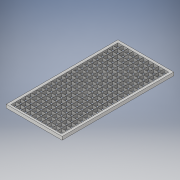
# Autodesk Inventor part: Lathhouse wall
Saved by Autodesk Inventor 2018 (Build 220112000, 112)
## iProperties
Created: 2019-05-08
Part Number: Lathhouse wall
Material: Generic
Document SubType Name: Modeling
Designer: 10043883
Density: 1 g/cm^3
Appearance: Default
Author: 10043883
Autodesk Inventor part; units mm, degrees
(part 1 of 2)
ref_plane "YZ Plane" through (0, 0, 0) normal (1, 0, 0) x (0, 1, 0)
ref_plane "XZ Plane" through (0, 0, 0) normal (0, 1, 0) x (-1, 0, 0)
ref_plane "XY Plane" through (0, 0, 0) normal (0, 0, 1) x (1, 0, 0)
sketch "Sketch1" plane through (0, 0, 0) normal (0, 1, 0) x (-1, 0, 0)
  line L0 (0, 0) -> (-3048, 0)
  line L1 (-3048, 0) -> (-3048, -6096)
  line L2 (-3048, -6096) -> (0, -6096)
  line L3 (0, -6096) -> (0, 0)
  dimension "d0" = 3048
  dimension "d1" = 6096
  constraints: 8 end point, 2 parallel, 1 horizontal, 1 perpendicular
  measures "d0" distance of L2.end L1.end
  measures "d1" distance of L1.end L0.end
extrude "Extrusion1" add sketch "Sketch1" along normal blind 177.8
sketch "Sketch2" plane through (0, 177.8, 0) normal (0, 1, 0) x (1, 0, 0)
  line L0 (146.7236, 110.4132) -> (400.7236, 110.4132)
  line L1 (400.7236, 110.4132) -> (400.7236, 364.4132)
  line L2 (400.7236, 364.4132) -> (146.7236, 364.4132)
  line L3 (146.7236, 364.4132) -> (146.7236, 110.4132)
  line L4 (146.7236, 110.4132) -> (400.7236, 364.4132) construction
  line L5 (400.7236, 110.4132) -> (146.7236, 364.4132) construction
  line L6 (400.7236, 110.4132) -> (3048, 110.4132) construction
  line L7 (3048, 0) -> (3048, 6096) construction
  line L8 (146.7236, 110.4132) -> (146.7236, 5658.2248) construction
  line L9 (146.7236, 389.8132) -> (400.7236, 389.8132)
  line L10 (400.7236, 389.8132) -> (400.7236, 643.8132)
  line L11 (400.7236, 643.8132) -> (146.7236, 643.8132)
  line L12 (146.7236, 643.8132) -> (146.7236, 389.8132)
  line L13 (146.7236, 669.2132) -> (400.7236, 669.2132)
  line L14 (400.7236, 669.2132) -> (400.7236, 923.2132)
  line L15 (400.7236, 923.2132) -> (146.7236, 923.2132)
  line L16 (146.7236, 923.2132) -> (146.7236, 669.2132)
  line L17 (146.7236, 948.6132) -> (400.7236, 948.6132)
  line L18 (400.7236, 948.6132) -> (400.7236, 1202.6132)
  line L19 (400.7236, 1202.6132) -> (146.7236, 1202.6132)
  line L20 (146.7236, 1202.6132) -> (146.7236, 948.6132)
  line L21 (146.7236, 1228.0132) -> (400.7236, 1228.0132)
  line L22 (400.7236, 1228.0132) -> (400.7236, 1482.0132)
  line L23 (400.7236, 1482.0132) -> (146.7236, 1482.0132)
  line L24 (146.7236, 1482.0132) -> (146.7236, 1228.0132)
  line L25 (146.7236, 1507.4132) -> (400.7236, 1507.4132)
  line L26 (400.7236, 1507.4132) -> (400.7236, 1761.4132)
  line L27 (400.7236, 1761.4132) -> (146.7236, 1761.4132)
  line L28 (146.7236, 1761.4132) -> (146.7236, 1507.4132)
  line L29 (146.7236, 1786.8132) -> (400.7236, 1786.8132)
  line L30 (400.7236, 1786.8132) -> (400.7236, 2040.8132)
  line L31 (400.7236, 2040.8132) -> (146.7236, 2040.8132)
  line L32 (146.7236, 2040.8132) -> (146.7236, 1786.8132)
  line L33 (146.7236, 2066.2132) -> (400.7236, 2066.2132)
  line L34 (400.7236, 2066.2132) -> (400.7236, 2320.2132)
  line L35 (400.7236, 2320.2132) -> (146.7236, 2320.2132)
  line L36 (146.7236, 2320.2132) -> (146.7236, 2066.2132)
  line L37 (146.7236, 2345.6132) -> (400.7236, 2345.6132)
  line L38 (400.7236, 2345.6132) -> (400.7236, 2599.6132)
  line L39 (400.7236, 2599.6132) -> (146.7236, 2599.6132)
  line L40 (146.7236, 2599.6132) -> (146.7236, 2345.6132)
  line L41 (146.7236, 2625.0132) -> (400.7236, 2625.0132)
  line L42 (400.7236, 2625.0132) -> (400.7236, 2879.0132)
  line L43 (400.7236, 2879.0132) -> (146.7236, 2879.0132)
  line L44 (146.7236, 2879.0132) -> (146.7236, 2625.0132)
  line L45 (146.7236, 2904.4132) -> (400.7236, 2904.4132)
  line L46 (400.7236, 2904.4132) -> (400.7236, 3158.4132)
  line L47 (400.7236, 3158.4132) -> (146.7236, 3158.4132)
  line L48 (146.7236, 3158.4132) -> (146.7236, 2904.4132)
  line L49 (146.7236, 3183.8132) -> (400.7236, 3183.8132)
  line L50 (400.7236, 3183.8132) -> (400.7236, 3437.8132)
  line L51 (400.7236, 3437.8132) -> (146.7236, 3437.8132)
  line L52 (146.7236, 3437.8132) -> (146.7236, 3183.8132)
  line L53 (146.7236, 3463.2132) -> (400.7236, 3463.2132)
  line L54 (400.7236, 3463.2132) -> (400.7236, 3717.2132)
  line L55 (400.7236, 3717.2132) -> (146.7236, 3717.2132)
  line L56 (146.7236, 3717.2132) -> (146.7236, 3463.2132)
  line L57 (146.7236, 3742.6132) -> (400.7236, 3742.6132)
  line L58 (400.7236, 3742.6132) -> (400.7236, 3996.6132)
  line L59 (400.7236, 3996.6132) -> (146.7236, 3996.6132)
  line L60 (146.7236, 3996.6132) -> (146.7236, 3742.6132)
  line L61 (146.7236, 4022.0132) -> (400.7236, 4022.0132)
  line L62 (400.7236, 4022.0132) -> (400.7236, 4276.0132)
  line L63 (400.7236, 4276.0132) -> (146.7236, 4276.0132)
  line L64 (146.7236, 4276.0132) -> (146.7236, 4022.0132)
  line L65 (146.7236, 4301.4132) -> (400.7236, 4301.4132)
  line L66 (400.7236, 4301.4132) -> (400.7236, 4555.4132)
  line L67 (400.7236, 4555.4132) -> (146.7236, 4555.4132)
  line L68 (146.7236, 4555.4132) -> (146.7236, 4301.4132)
  line L69 (146.7236, 4580.8132) -> (400.7236, 4580.8132)
  line L70 (400.7236, 4580.8132) -> (400.7236, 4834.8132)
  line L71 (400.7236, 4834.8132) -> (146.7236, 4834.8132)
  line L72 (146.7236, 4834.8132) -> (146.7236, 4580.8132)
  line L73 (146.7236, 4860.2132) -> (400.7236, 4860.2132)
  line L74 (400.7236, 4860.2132) -> (400.7236, 5114.2132)
  line L75 (400.7236, 5114.2132) -> (146.7236, 5114.2132)
  line L76 (146.7236, 5114.2132) -> (146.7236, 4860.2132)
  line L77 (146.7236, 5139.6132) -> (400.7236, 5139.6132)
  line L78 (400.7236, 5139.6132) -> (400.7236, 5393.6132)
  line L79 (400.7236, 5393.6132) -> (146.7236, 5393.6132)
  line L80 (146.7236, 5393.6132) -> (146.7236, 5139.6132)
  line L81 (146.7236, 5419.0132) -> (400.7236, 5419.0132)
  line L82 (400.7236, 5419.0132) -> (400.7236, 5673.0132)
  line L83 (400.7236, 5673.0132) -> (146.7236, 5673.0132)
  line L84 (146.7236, 5673.0132) -> (146.7236, 5419.0132)
  line L85 (146.7236, 5698.4132) -> (400.7236, 5698.4132)
  line L86 (400.7236, 5698.4132) -> (400.7236, 5952.4132)
  line L87 (400.7236, 5952.4132) -> (146.7236, 5952.4132)
  line L88 (146.7236, 5952.4132) -> (146.7236, 5698.4132)
  line L89 (426.1236, 110.4132) -> (680.1236, 110.4132)
  line L90 (680.1236, 110.4132) -> (680.1236, 364.4132)
  line L91 (680.1236, 364.4132) -> (426.1236, 364.4132)
  line L92 (426.1236, 364.4132) -> (426.1236, 110.4132)
  line L93 (426.1236, 389.8132) -> (680.1236, 389.8132)
  line L94 (680.1236, 389.8132) -> (680.1236, 643.8132)
  line L95 (680.1236, 643.8132) -> (426.1236, 643.8132)
  line L96 (426.1236, 643.8132) -> (426.1236, 389.8132)
  line L97 (426.1236, 669.2132) -> (680.1236, 669.2132)
  line L98 (680.1236, 669.2132) -> (680.1236, 923.2132)
  line L99 (680.1236, 923.2132) -> (426.1236, 923.2132)
  line L100 (426.1236, 923.2132) -> (426.1236, 669.2132)
  line L101 (426.1236, 948.6132) -> (680.1236, 948.6132)
  line L102 (680.1236, 948.6132) -> (680.1236, 1202.6132)
  line L103 (680.1236, 1202.6132) -> (426.1236, 1202.6132)
  line L104 (426.1236, 1202.6132) -> (426.1236, 948.6132)
  line L105 (426.1236, 1228.0132) -> (680.1236, 1228.0132)
  line L106 (680.1236, 1228.0132) -> (680.1236, 1482.0132)
  line L107 (680.1236, 1482.0132) -> (426.1236, 1482.0132)
  line L108 (426.1236, 1482.0132) -> (426.1236, 1228.0132)
  line L109 (426.1236, 1507.4132) -> (680.1236, 1507.4132)
  line L110 (680.1236, 1507.4132) -> (680.1236, 1761.4132)
  line L111 (680.1236, 1761.4132) -> (426.1236, 1761.4132)
  line L112 (426.1236, 1761.4132) -> (426.1236, 1507.4132)
  line L113 (426.1236, 1786.8132) -> (680.1236, 1786.8132)
  line L114 (680.1236, 1786.8132) -> (680.1236, 2040.8132)
  line L115 (680.1236, 2040.8132) -> (426.1236, 2040.8132)
  line L116 (426.1236, 2040.8132) -> (426.1236, 1786.8132)
  line L117 (426.1236, 2066.2132) -> (680.1236, 2066.2132)
  line L118 (680.1236, 2066.2132) -> (680.1236, 2320.2132)
  line L119 (680.1236, 2320.2132) -> (426.1236, 2320.2132)
  line L120 (426.1236, 2320.2132) -> (426.1236, 2066.2132)
  line L121 (426.1236, 2345.6132) -> (680.1236, 2345.6132)
  line L122 (680.1236, 2345.6132) -> (680.1236, 2599.6132)
  line L123 (680.1236, 2599.6132) -> (426.1236, 2599.6132)
  line L124 (426.1236, 2599.6132) -> (426.1236, 2345.6132)
  line L125 (426.1236, 2625.0132) -> (680.1236, 2625.0132)
  line L126 (680.1236, 2625.0132) -> (680.1236, 2879.0132)
  line L127 (680.1236, 2879.0132) -> (426.1236, 2879.0132)
  line L128 (426.1236, 2879.0132) -> (426.1236, 2625.0132)
  line L129 (426.1236, 2904.4132) -> (680.1236, 2904.4132)
  line L130 (680.1236, 2904.4132) -> (680.1236, 3158.4132)
  line L131 (680.1236, 3158.4132) -> (426.1236, 3158.4132)
  line L132 (426.1236, 3158.4132) -> (426.1236, 2904.4132)
  line L133 (426.1236, 3183.8132) -> (680.1236, 3183.8132)
  line L134 (680.1236, 3183.8132) -> (680.1236, 3437.8132)
  line L135 (680.1236, 3437.8132) -> (426.1236, 3437.8132)
  line L136 (426.1236, 3437.8132) -> (426.1236, 3183.8132)
  line L137 (426.1236, 3463.2132) -> (680.1236, 3463.2132)
  line L138 (680.1236, 3463.2132) -> (680.1236, 3717.2132)
  line L139 (680.1236, 3717.2132) -> (426.1236, 3717.2132)
  line L140 (426.1236, 3717.2132) -> (426.1236, 3463.2132)
  line L141 (426.1236, 3742.6132) -> (680.1236, 3742.6132)
  line L142 (680.1236, 3742.6132) -> (680.1236, 3996.6132)
  line L143 (680.1236, 3996.6132) -> (426.1236, 3996.6132)
  line L144 (426.1236, 3996.6132) -> (426.1236, 3742.6132)
  line L145 (426.1236, 4022.0132) -> (680.1236, 4022.0132)
  line L146 (680.1236, 4022.0132) -> (680.1236, 4276.0132)
  line L147 (680.1236, 4276.0132) -> (426.1236, 4276.0132)
  line L148 (426.1236, 4276.0132) -> (426.1236, 4022.0132)
  line L149 (426.1236, 4301.4132) -> (680.1236, 4301.4132)
  line L150 (680.1236, 4301.4132) -> (680.1236, 4555.4132)
  line L151 (680.1236, 4555.4132) -> (426.1236, 4555.4132)
  line L152 (426.1236, 4555.4132) -> (426.1236, 4301.4132)
  line L153 (426.1236, 4580.8132) -> (680.1236, 4580.8132)
  line L154 (680.1236, 4580.8132) -> (680.1236, 4834.8132)
  line L155 (680.1236, 4834.8132) -> (426.1236, 4834.8132)
  line L156 (426.1236, 4834.8132) -> (426.1236, 4580.8132)
  line L157 (426.1236, 4860.2132) -> (680.1236, 4860.2132)
  line L158 (680.1236, 4860.2132) -> (680.1236, 5114.2132)
  line L159 (680.1236, 5114.2132) -> (426.1236, 5114.2132)
  line L160 (426.1236, 5114.2132) -> (426.1236, 4860.2132)
  line L161 (426.1236, 5139.6132) -> (680.1236, 5139.6132)
  line L162 (680.1236, 5139.6132) -> (680.1236, 5393.6132)
  line L163 (680.1236, 5393.6132) -> (426.1236, 5393.6132)
  line L164 (426.1236, 5393.6132) -> (426.1236, 5139.6132)
  line L165 (426.1236, 5419.0132) -> (680.1236, 5419.0132)
  line L166 (680.1236, 5419.0132) -> (680.1236, 5673.0132)
  line L167 (680.1236, 5673.0132) -> (426.1236, 5673.0132)
  line L168 (426.1236, 5673.0132) -> (426.1236, 5419.0132)
  line L169 (426.1236, 5698.4132) -> (680.1236, 5698.4132)
  line L170 (680.1236, 5698.4132) -> (680.1236, 5952.4132)
  line L171 (680.1236, 5952.4132) -> (426.1236, 5952.4132)
  line L172 (426.1236, 5952.4132) -> (426.1236, 5698.4132)
  line L173 (705.5236, 110.4132) -> (959.5236, 110.4132)
  line L174 (959.5236, 110.4132) -> (959.5236, 364.4132)
  line L175 (959.5236, 364.4132) -> (705.5236, 364.4132)
  line L176 (705.5236, 364.4132) -> (705.5236, 110.4132)
  line L177 (705.5236, 389.8132) -> (959.5236, 389.8132)
  line L178 (959.5236, 389.8132) -> (959.5236, 643.8132)
  line L179 (959.5236, 643.8132) -> (705.5236, 643.8132)
  line L180 (705.5236, 643.8132) -> (705.5236, 389.8132)
  line L181 (705.5236, 669.2132) -> (959.5236, 669.2132)
  line L182 (959.5236, 669.2132) -> (959.5236, 923.2132)
  line L183 (959.5236, 923.2132) -> (705.5236, 923.2132)
  line L184 (705.5236, 923.2132) -> (705.5236, 669.2132)
  line L185 (705.5236, 948.6132) -> (959.5236, 948.6132)
  line L186 (959.5236, 948.6132) -> (959.5236, 1202.6132)
  line L187 (959.5236, 1202.6132) -> (705.5236, 1202.6132)
  line L188 (705.5236, 1202.6132) -> (705.5236, 948.6132)
  line L189 (705.5236, 1228.0132) -> (959.5236, 1228.0132)
  line L190 (959.5236, 1228.0132) -> (959.5236, 1482.0132)
  line L191 (959.5236, 1482.0132) -> (705.5236, 1482.0132)
  line L192 (705.5236, 1482.0132) -> (705.5236, 1228.0132)
  line L193 (705.5236, 1507.4132) -> (959.5236, 1507.4132)
  line L194 (959.5236, 1507.4132) -> (959.5236, 1761.4132)
  line L195 (959.5236, 1761.4132) -> (705.5236, 1761.4132)
  line L196 (705.5236, 1761.4132) -> (705.5236, 1507.4132)
  line L197 (705.5236, 1786.8132) -> (959.5236, 1786.8132)
  line L198 (959.5236, 1786.8132) -> (959.5236, 2040.8132)
  line L199 (959.5236, 2040.8132) -> (705.5236, 2040.8132)
  line L200 (705.5236, 2040.8132) -> (705.5236, 1786.8132)
  line L201 (705.5236, 2066.2132) -> (959.5236, 2066.2132)
  line L202 (959.5236, 2066.2132) -> (959.5236, 2320.2132)
  line L203 (959.5236, 2320.2132) -> (705.5236, 2320.2132)
  line L204 (705.5236, 2320.2132) -> (705.5236, 2066.2132)
  line L205 (705.5236, 2345.6132) -> (959.5236, 2345.6132)
  line L206 (959.5236, 2345.6132) -> (959.5236, 2599.6132)
  line L207 (959.5236, 2599.6132) -> (705.5236, 2599.6132)
  line L208 (705.5236, 2599.6132) -> (705.5236, 2345.6132)
  line L209 (705.5236, 2625.0132) -> (959.5236, 2625.0132)
  line L210 (959.5236, 2625.0132) -> (959.5236, 2879.0132)
  line L211 (959.5236, 2879.0132) -> (705.5236, 2879.0132)
  line L212 (705.5236, 2879.0132) -> (705.5236, 2625.0132)
  line L213 (705.5236, 2904.4132) -> (959.5236, 2904.4132)
  line L214 (959.5236, 2904.4132) -> (959.5236, 3158.4132)
  line L215 (959.5236, 3158.4132) -> (705.5236, 3158.4132)
  line L216 (705.5236, 3158.4132) -> (705.5236, 2904.4132)
  line L217 (705.5236, 3183.8132) -> (959.5236, 3183.8132)
  line L218 (959.5236, 3183.8132) -> (959.5236, 3437.8132)
  line L219 (959.5236, 3437.8132) -> (705.5236, 3437.8132)
  line L220 (705.5236, 3437.8132) -> (705.5236, 3183.8132)
  line L221 (705.5236, 3463.2132) -> (959.5236, 3463.2132)
  line L222 (959.5236, 3463.2132) -> (959.5236, 3717.2132)
  line L223 (959.5236, 3717.2132) -> (705.5236, 3717.2132)
  line L224 (705.5236, 3717.2132) -> (705.5236, 3463.2132)
  line L225 (705.5236, 3742.6132) -> (959.5236, 3742.6132)
  line L226 (959.5236, 3742.6132) -> (959.5236, 3996.6132)
  line L227 (959.5236, 3996.6132) -> (705.5236, 3996.6132)
  line L228 (705.5236, 3996.6132) -> (705.5236, 3742.6132)
  line L229 (705.5236, 4022.0132) -> (959.5236, 4022.0132)
  line L230 (959.5236, 4022.0132) -> (959.5236, 4276.0132)
  line L231 (959.5236, 4276.0132) -> (705.5236, 4276.0132)
  line L232 (705.5236, 4276.0132) -> (705.5236, 4022.0132)
  line L233 (705.5236, 4301.4132) -> (959.5236, 4301.4132)
  line L234 (959.5236, 4301.4132) -> (959.5236, 4555.4132)
  line L235 (959.5236, 4555.4132) -> (705.5236, 4555.4132)
  line L236 (705.5236, 4555.4132) -> (705.5236, 4301.4132)
  line L237 (705.5236, 4580.8132) -> (959.5236, 4580.8132)
  line L238 (959.5236, 4580.8132) -> (959.5236, 4834.8132)
  line L239 (959.5236, 4834.8132) -> (705.5236, 4834.8132)
  line L240 (705.5236, 4834.8132) -> (705.5236, 4580.8132)
  line L241 (705.5236, 4860.2132) -> (959.5236, 4860.2132)
  line L242 (959.5236, 4860.2132) -> (959.5236, 5114.2132)
  line L243 (959.5236, 5114.2132) -> (705.5236, 5114.2132)
  line L244 (705.5236, 5114.2132) -> (705.5236, 4860.2132)
  line L245 (705.5236, 5139.6132) -> (959.5236, 5139.6132)
  line L246 (959.5236, 5139.6132) -> (959.5236, 5393.6132)
  line L247 (959.5236, 5393.6132) -> (705.5236, 5393.6132)
  line L248 (705.5236, 5393.6132) -> (705.5236, 5139.6132)
  line L249 (705.5236, 5419.0132) -> (959.5236, 5419.0132)
  line L250 (959.5236, 5419.0132) -> (959.5236, 5673.0132)
  line L251 (959.5236, 5673.0132) -> (705.5236, 5673.0132)
  line L252 (705.5236, 5673.0132) -> (705.5236, 5419.0132)
  line L253 (705.5236, 5698.4132) -> (959.5236, 5698.4132)
  line L254 (959.5236, 5698.4132) -> (959.5236, 5952.4132)
  line L255 (959.5236, 5952.4132) -> (705.5236, 5952.4132)
  line L256 (705.5236, 5952.4132) -> (705.5236, 5698.4132)
  line L257 (984.9236, 110.4132) -> (1238.9236, 110.4132)
  line L258 (1238.9236, 110.4132) -> (1238.9236, 364.4132)
  line L259 (1238.9236, 364.4132) -> (984.9236, 364.4132)
  line L260 (984.9236, 364.4132) -> (984.9236, 110.4132)
  line L261 (984.9236, 389.8132) -> (1238.9236, 389.8132)
  line L262 (1238.9236, 389.8132) -> (1238.9236, 643.8132)
  line L263 (1238.9236, 643.8132) -> (984.9236, 643.8132)
  line L264 (984.9236, 643.8132) -> (984.9236, 389.8132)
  line L265 (984.9236, 669.2132) -> (1238.9236, 669.2132)
  line L266 (1238.9236, 669.2132) -> (1238.9236, 923.2132)
  line L267 (1238.9236, 923.2132) -> (984.9236, 923.2132)
  line L268 (984.9236, 923.2132) -> (984.9236, 669.2132)
  line L269 (984.9236, 948.6132) -> (1238.9236, 948.6132)
  line L270 (1238.9236, 948.6132) -> (1238.9236, 1202.6132)
  line L271 (1238.9236, 1202.6132) -> (984.9236, 1202.6132)
  line L272 (984.9236, 1202.6132) -> (984.9236, 948.6132)
  line L273 (984.9236, 1228.0132) -> (1238.9236, 1228.0132)
  line L274 (1238.9236, 1228.0132) -> (1238.9236, 1482.0132)
  line L275 (1238.9236, 1482.0132) -> (984.9236, 1482.0132)
  line L276 (984.9236, 1482.0132) -> (984.9236, 1228.0132)
  line L277 (984.9236, 1507.4132) -> (1238.9236, 1507.4132)
  line L278 (1238.9236, 1507.4132) -> (1238.9236, 1761.4132)
  line L279 (1238.9236, 1761.4132) -> (984.9236, 1761.4132)
  line L280 (984.9236, 1761.4132) -> (984.9236, 1507.4132)
  line L281 (984.9236, 1786.8132) -> (1238.9236, 1786.8132)
  line L282 (1238.9236, 1786.8132) -> (1238.9236, 2040.8132)
  line L283 (1238.9236, 2040.8132) -> (984.9236, 2040.8132)
  line L284 (984.9236, 2040.8132) -> (984.9236, 1786.8132)
  line L285 (984.9236, 2066.2132) -> (1238.9236, 2066.2132)
  line L286 (1238.9236, 2066.2132) -> (1238.9236, 2320.2132)
  line L287 (1238.9236, 2320.2132) -> (984.9236, 2320.2132)
  line L288 (984.9236, 2320.2132) -> (984.9236, 2066.2132)
  line L289 (984.9236, 2345.6132) -> (1238.9236, 2345.6132)
  line L290 (1238.9236, 2345.6132) -> (1238.9236, 2599.6132)
  line L291 (1238.9236, 2599.6132) -> (984.9236, 2599.6132)
  line L292 (984.9236, 2599.6132) -> (984.9236, 2345.6132)
  line L293 (984.9236, 2625.0132) -> (1238.9236, 2625.0132)
  line L294 (1238.9236, 2625.0132) -> (1238.9236, 2879.0132)
  line L295 (1238.9236, 2879.0132) -> (984.9236, 2879.0132)
  line L296 (984.9236, 2879.0132) -> (984.9236, 2625.0132)
  line L297 (984.9236, 2904.4132) -> (1238.9236, 2904.4132)
  line L298 (1238.9236, 2904.4132) -> (1238.9236, 3158.4132)
  line L299 (1238.9236, 3158.4132) -> (984.9236, 3158.4132)
  line L300 (984.9236, 3158.4132) -> (984.9236, 2904.4132)
  line L301 (984.9236, 3183.8132) -> (1238.9236, 3183.8132)
  line L302 (1238.9236, 3183.8132) -> (1238.9236, 3437.8132)
  line L303 (1238.9236, 3437.8132) -> (984.9236, 3437.8132)
  line L304 (984.9236, 3437.8132) -> (984.9236, 3183.8132)
  line L305 (984.9236, 3463.2132) -> (1238.9236, 3463.2132)
  line L306 (1238.9236, 3463.2132) -> (1238.9236, 3717.2132)
  line L307 (1238.9236, 3717.2132) -> (984.9236, 3717.2132)
  line L308 (984.9236, 3717.2132) -> (984.9236, 3463.2132)
  line L309 (984.9236, 3742.6132) -> (1238.9236, 3742.6132)
  line L310 (1238.9236, 3742.6132) -> (1238.9236, 3996.6132)
  line L311 (1238.9236, 3996.6132) -> (984.9236, 3996.6132)
  line L312 (984.9236, 3996.6132) -> (984.9236, 3742.6132)
  line L313 (984.9236, 4022.0132) -> (1238.9236, 4022.0132)
  line L314 (1238.9236, 4022.0132) -> (1238.9236, 4276.0132)
  line L315 (1238.9236, 4276.0132) -> (984.9236, 4276.0132)
  line L316 (984.9236, 4276.0132) -> (984.9236, 4022.0132)
  line L317 (984.9236, 4301.4132) -> (1238.9236, 4301.4132)
  line L318 (1238.9236, 4301.4132) -> (1238.9236, 4555.4132)
  line L319 (1238.9236, 4555.4132) -> (984.9236, 4555.4132)
  line L320 (984.9236, 4555.4132) -> (984.9236, 4301.4132)
  line L321 (984.9236, 4580.8132) -> (1238.9236, 4580.8132)
  line L322 (1238.9236, 4580.8132) -> (1238.9236, 4834.8132)
  line L323 (1238.9236, 4834.8132) -> (984.9236, 4834.8132)
  line L324 (984.9236, 4834.8132) -> (984.9236, 4580.8132)
  line L325 (984.9236, 4860.2132) -> (1238.9236, 4860.2132)
  line L326 (1238.9236, 4860.2132) -> (1238.9236, 5114.2132)
  line L327 (1238.9236, 5114.2132) -> (984.9236, 5114.2132)
  line L328 (984.9236, 5114.2132) -> (984.9236, 4860.2132)
  line L329 (984.9236, 5139.6132) -> (1238.9236, 5139.6132)
  line L330 (1238.9236, 5139.6132) -> (1238.9236, 5393.6132)
  line L331 (1238.9236, 5393.6132) -> (984.9236, 5393.6132)
  line L332 (984.9236, 5393.6132) -> (984.9236, 5139.6132)
  line L333 (984.9236, 5419.0132) -> (1238.9236, 5419.0132)
  line L334 (1238.9236, 5419.0132) -> (1238.9236, 5673.0132)
  line L335 (1238.9236, 5673.0132) -> (984.9236, 5673.0132)
  line L336 (984.9236, 5673.0132) -> (984.9236, 5419.0132)
  line L337 (984.9236, 5698.4132) -> (1238.9236, 5698.4132)
  line L338 (1238.9236, 5698.4132) -> (1238.9236, 5952.4132)
  line L339 (1238.9236, 5952.4132) -> (984.9236, 5952.4132)
  line L340 (984.9236, 5952.4132) -> (984.9236, 5698.4132)
  line L341 (1264.3236, 110.4132) -> (1518.3236, 110.4132)
  line L342 (1518.3236, 110.4132) -> (1518.3236, 364.4132)
  line L343 (1518.3236, 364.4132) -> (1264.3236, 364.4132)
  line L344 (1264.3236, 364.4132) -> (1264.3236, 110.4132)
  line L345 (1264.3236, 389.8132) -> (1518.3236, 389.8132)
  line L346 (1518.3236, 389.8132) -> (1518.3236, 643.8132)
  line L347 (1518.3236, 643.8132) -> (1264.3236, 643.8132)
  line L348 (1264.3236, 643.8132) -> (1264.3236, 389.8132)
  line L349 (1264.3236, 669.2132) -> (1518.3236, 669.2132)
  line L350 (1518.3236, 669.2132) -> (1518.3236, 923.2132)
  line L351 (1518.3236, 923.2132) -> (1264.3236, 923.2132)
  line L352 (1264.3236, 923.2132) -> (1264.3236, 669.2132)
  line L353 (1264.3236, 948.6132) -> (1518.3236, 948.6132)
  line L354 (1518.3236, 948.6132) -> (1518.3236, 1202.6132)
  line L355 (1518.3236, 1202.6132) -> (1264.3236, 1202.6132)
  line L356 (1264.3236, 1202.6132) -> (1264.3236, 948.6132)
  line L357 (1264.3236, 1228.0132) -> (1518.3236, 1228.0132)
  line L358 (1518.3236, 1228.0132) -> (1518.3236, 1482.0132)
  line L359 (1518.3236, 1482.0132) -> (1264.3236, 1482.0132)
  line L360 (1264.3236, 1482.0132) -> (1264.3236, 1228.0132)
  line L361 (1264.3236, 1507.4132) -> (1518.3236, 1507.4132)
  line L362 (1518.3236, 1507.4132) -> (1518.3236, 1761.4132)
  line L363 (1518.3236, 1761.4132) -> (1264.3236, 1761.4132)
  line L364 (1264.3236, 1761.4132) -> (1264.3236, 1507.4132)
  line L365 (1264.3236, 1786.8132) -> (1518.3236, 1786.8132)
  line L366 (1518.3236, 1786.8132) -> (1518.3236, 2040.8132)
  line L367 (1518.3236, 2040.8132) -> (1264.3236, 2040.8132)
  line L368 (1264.3236, 2040.8132) -> (1264.3236, 1786.8132)
  line L369 (1264.3236, 2066.2132) -> (1518.3236, 2066.2132)
  line L370 (1518.3236, 2066.2132) -> (1518.3236, 2320.2132)
  line L371 (1518.3236, 2320.2132) -> (1264.3236, 2320.2132)
  line L372 (1264.3236, 2320.2132) -> (1264.3236, 2066.2132)
  line L373 (1264.3236, 2345.6132) -> (1518.3236, 2345.6132)
  line L374 (1518.3236, 2345.6132) -> (1518.3236, 2599.6132)
  line L375 (1518.3236, 2599.6132) -> (1264.3236, 2599.6132)
  line L376 (1264.3236, 2599.6132) -> (1264.3236, 2345.6132)
  line L377 (1264.3236, 2625.0132) -> (1518.3236, 2625.0132)
  line L378 (1518.3236, 2625.0132) -> (1518.3236, 2879.0132)
  line L379 (1518.3236, 2879.0132) -> (1264.3236, 2879.0132)
  line L380 (1264.3236, 2879.0132) -> (1264.3236, 2625.0132)
  line L381 (1264.3236, 2904.4132) -> (1518.3236, 2904.4132)
  line L382 (1518.3236, 2904.4132) -> (1518.3236, 3158.4132)
  line L383 (1518.3236, 3158.4132) -> (1264.3236, 3158.4132)
  line L384 (1264.3236, 3158.4132) -> (1264.3236, 2904.4132)
  line L385 (1264.3236, 3183.8132) -> (1518.3236, 3183.8132)
  line L386 (1518.3236, 3183.8132) -> (1518.3236, 3437.8132)
  line L387 (1518.3236, 3437.8132) -> (1264.3236, 3437.8132)
  line L388 (1264.3236, 3437.8132) -> (1264.3236, 3183.8132)
  line L389 (1264.3236, 3463.2132) -> (1518.3236, 3463.2132)
  line L390 (1518.3236, 3463.2132) -> (1518.3236, 3717.2132)
  line L391 (1518.3236, 3717.2132) -> (1264.3236, 3717.2132)
  line L392 (1264.3236, 3717.2132) -> (1264.3236, 3463.2132)
  line L393 (1264.3236, 3742.6132) -> (1518.3236, 3742.6132)
  line L394 (1518.3236, 3742.6132) -> (1518.3236, 3996.6132)
  line L395 (1518.3236, 3996.6132) -> (1264.3236, 3996.6132)
  line L396 (1264.3236, 3996.6132) -> (1264.3236, 3742.6132)
  line L397 (1264.3236, 4022.0132) -> (1518.3236, 4022.0132)
  line L398 (1518.3236, 4022.0132) -> (1518.3236, 4276.0132)
  line L399 (1518.3236, 4276.0132) -> (1264.3236, 4276.0132)
  line L400 (1264.3236, 4276.0132) -> (1264.3236, 4022.0132)
  line L401 (1264.3236, 4301.4132) -> (1518.3236, 4301.4132)
  line L402 (1518.3236, 4301.4132) -> (1518.3236, 4555.4132)
  line L403 (1518.3236, 4555.4132) -> (1264.3236, 4555.4132)
  line L404 (1264.3236, 4555.4132) -> (1264.3236, 4301.4132)
  line L405 (1264.3236, 4580.8132) -> (1518.3236, 4580.8132)
  line L406 (1518.3236, 4580.8132) -> (1518.3236, 4834.8132)
  line L407 (1518.3236, 4834.8132) -> (1264.3236, 4834.8132)
  line L408 (1264.3236, 4834.8132) -> (1264.3236, 4580.8132)
  line L409 (1264.3236, 4860.2132) -> (1518.3236, 4860.2132)
  line L410 (1518.3236, 4860.2132) -> (1518.3236, 5114.2132)
  line L411 (1518.3236, 5114.2132) -> (1264.3236, 5114.2132)
  line L412 (1264.3236, 5114.2132) -> (1264.3236, 4860.2132)
  line L413 (1264.3236, 5139.6132) -> (1518.3236, 5139.6132)
  line L414 (1518.3236, 5139.6132) -> (1518.3236, 5393.6132)
  line L415 (1518.3236, 5393.6132) -> (1264.3236, 5393.6132)
  line L416 (1264.3236, 5393.6132) -> (1264.3236, 5139.6132)
  line L417 (1264.3236, 5419.0132) -> (1518.3236, 5419.0132)
  line L418 (1518.3236, 5419.0132) -> (1518.3236, 5673.0132)
  line L419 (1518.3236, 5673.0132) -> (1264.3236, 5673.0132)
  line L420 (1264.3236, 5673.0132) -> (1264.3236, 5419.0132)
  line L421 (1264.3236, 5698.4132) -> (1518.3236, 5698.4132)
  line L422 (1518.3236, 5698.4132) -> (1518.3236, 5952.4132)
  line L423 (1518.3236, 5952.4132) -> (1264.3236, 5952.4132)
  line L424 (1264.3236, 5952.4132) -> (1264.3236, 5698.4132)
  line L425 (1543.7236, 110.4132) -> (1797.7236, 110.4132)
  line L426 (1797.7236, 110.4132) -> (1797.7236, 364.4132)
  line L427 (1797.7236, 364.4132) -> (1543.7236, 364.4132)
  line L428 (1543.7236, 364.4132) -> (1543.7236, 110.4132)
  line L429 (1543.7236, 389.8132) -> (1797.7236, 389.8132)
  line L430 (1797.7236, 389.8132) -> (1797.7236, 643.8132)
  line L431 (1797.7236, 643.8132) -> (1543.7236, 643.8132)
  line L432 (1543.7236, 643.8132) -> (1543.7236, 389.8132)
  line L433 (1543.7236, 669.2132) -> (1797.7236, 669.2132)
  line L434 (1797.7236, 669.2132) -> (1797.7236, 923.2132)
  line L435 (1797.7236, 923.2132) -> (1543.7236, 923.2132)
  line L436 (1543.7236, 923.2132) -> (1543.7236, 669.2132)
  line L437 (1543.7236, 948.6132) -> (1797.7236, 948.6132)
  line L438 (1797.7236, 948.6132) -> (1797.7236, 1202.6132)
  line L439 (1797.7236, 1202.6132) -> (1543.7236, 1202.6132)
  line L440 (1543.7236, 1202.6132) -> (1543.7236, 948.6132)
  line L441 (1543.7236, 1228.0132) -> (1797.7236, 1228.0132)
  line L442 (1797.7236, 1228.0132) -> (1797.7236, 1482.0132)
  line L443 (1797.7236, 1482.0132) -> (1543.7236, 1482.0132)
  line L444 (1543.7236, 1482.0132) -> (1543.7236, 1228.0132)
  line L445 (1543.7236, 1507.4132) -> (1797.7236, 1507.4132)
  line L446 (1797.7236, 1507.4132) -> (1797.7236, 1761.4132)
  line L447 (1797.7236, 1761.4132) -> (1543.7236, 1761.4132)
  line L448 (1543.7236, 1761.4132) -> (1543.7236, 1507.4132)
  line L449 (1543.7236, 1786.8132) -> (1797.7236, 1786.8132)
  line L450 (1797.7236, 1786.8132) -> (1797.7236, 2040.8132)
  line L451 (1797.7236, 2040.8132) -> (1543.7236, 2040.8132)
  line L452 (1543.7236, 2040.8132) -> (1543.7236, 1786.8132)
  line L453 (1543.7236, 2066.2132) -> (1797.7236, 2066.2132)
  line L454 (1797.7236, 2066.2132) -> (1797.7236, 2320.2132)
  line L455 (1797.7236, 2320.2132) -> (1543.7236, 2320.2132)
  line L456 (1543.7236, 2320.2132) -> (1543.7236, 2066.2132)
  line L457 (1543.7236, 2345.6132) -> (1797.7236, 2345.6132)
  line L458 (1797.7236, 2345.6132) -> (1797.7236, 2599.6132)
  line L459 (1797.7236, 2599.6132) -> (1543.7236, 2599.6132)
  line L460 (1543.7236, 2599.6132) -> (1543.7236, 2345.6132)
  line L461 (1543.7236, 2625.0132) -> (1797.7236, 2625.0132)
  line L462 (1797.7236, 2625.0132) -> (1797.7236, 2879.0132)
  line L463 (1797.7236, 2879.0132) -> (1543.7236, 2879.0132)
  line L464 (1543.7236, 2879.0132) -> (1543.7236, 2625.0132)
  line L465 (1543.7236, 2904.4132) -> (1797.7236, 2904.4132)
  line L466 (1797.7236, 2904.4132) -> (1797.7236, 3158.4132)
  line L467 (1797.7236, 3158.4132) -> (1543.7236, 3158.4132)
  line L468 (1543.7236, 3158.4132) -> (1543.7236, 2904.4132)
  line L469 (1543.7236, 3183.8132) -> (1797.7236, 3183.8132)
  line L470 (1797.7236, 3183.8132) -> (1797.7236, 3437.8132)
  line L471 (1797.7236, 3437.8132) -> (1543.7236, 3437.8132)
  line L472 (1543.7236, 3437.8132) -> (1543.7236, 3183.8132)
  line L473 (1543.7236, 3463.2132) -> (1797.7236, 3463.2132)
  line L474 (1797.7236, 3463.2132) -> (1797.7236, 3717.2132)
  line L475 (1797.7236, 3717.2132) -> (1543.7236, 3717.2132)
  line L476 (1543.7236, 3717.2132) -> (1543.7236, 3463.2132)
  line L477 (1543.7236, 3742.6132) -> (1797.7236, 3742.6132)
  line L478 (1797.7236, 3742.6132) -> (1797.7236, 3996.6132)
  line L479 (1797.7236, 3996.6132) -> (1543.7236, 3996.6132)
  line L480 (1543.7236, 3996.6132) -> (1543.7236, 3742.6132)
  line L481 (1543.7236, 4022.0132) -> (1797.7236, 4022.0132)
  line L482 (1797.7236, 4022.0132) -> (1797.7236, 4276.0132)
  line L483 (1797.7236, 4276.0132) -> (1543.7236, 4276.0132)
  line L484 (1543.7236, 4276.0132) -> (1543.7236, 4022.0132)
  line L485 (1543.7236, 4301.4132) -> (1797.7236, 4301.4132)
  line L486 (1797.7236, 4301.4132) -> (1797.7236, 4555.4132)
  line L487 (1797.7236, 4555.4132) -> (1543.7236, 4555.4132)
  line L488 (1543.7236, 4555.4132) -> (1543.7236, 4301.4132)
  line L489 (1543.7236, 4580.8132) -> (1797.7236, 4580.8132)
  line L490 (1797.7236, 4580.8132) -> (1797.7236, 4834.8132)
  line L491 (1797.7236, 4834.8132) -> (1543.7236, 4834.8132)
  line L492 (1543.7236, 4834.8132) -> (1543.7236, 4580.8132)
  line L493 (1543.7236, 4860.2132) -> (1797.7236, 4860.2132)
  line L494 (1797.7236, 4860.2132) -> (1797.7236, 5114.2132)
  line L495 (1797.7236, 5114.2132) -> (1543.7236, 5114.2132)
  line L496 (1543.7236, 5114.2132) -> (1543.7236, 4860.2132)
  line L497 (1543.7236, 5139.6132) -> (1797.7236, 5139.6132)
  line L498 (1797.7236, 5139.6132) -> (1797.7236, 5393.6132)
  line L499 (1797.7236, 5393.6132) -> (1543.7236, 5393.6132)
  line L500 (1543.7236, 5393.6132) -> (1543.7236, 5139.6132)
  line L501 (1543.7236, 5419.0132) -> (1797.7236, 5419.0132)
  line L502 (1797.7236, 5419.0132) -> (1797.7236, 5673.0132)
  line L503 (1797.7236, 5673.0132) -> (1543.7236, 5673.0132)
  line L504 (1543.7236, 5673.0132) -> (1543.7236, 5419.0132)
  line L505 (1543.7236, 5698.4132) -> (1797.7236, 5698.4132)
  line L506 (1797.7236, 5698.4132) -> (1797.7236, 5952.4132)
  line L507 (1797.7236, 5952.4132) -> (1543.7236, 5952.4132)
  line L508 (1543.7236, 5952.4132) -> (1543.7236, 5698.4132)
  line L509 (1823.1236, 110.4132) -> (2077.1236, 110.4132)
  line L510 (2077.1236, 110.4132) -> (2077.1236, 364.4132)
  line L511 (2077.1236, 364.4132) -> (1823.1236, 364.4132)
  line L512 (1823.1236, 364.4132) -> (1823.1236, 110.4132)
  line L513 (1823.1236, 389.8132) -> (2077.1236, 389.8132)
  line L514 (2077.1236, 389.8132) -> (2077.1236, 643.8132)
  line L515 (2077.1236, 643.8132) -> (1823.1236, 643.8132)
  line L516 (1823.1236, 643.8132) -> (1823.1236, 389.8132)
  line L517 (1823.1236, 669.2132) -> (2077.1236, 669.2132)
  line L518 (2077.1236, 669.2132) -> (2077.1236, 923.2132)
  line L519 (2077.1236, 923.2132) -> (1823.1236, 923.2132)
  line L520 (1823.1236, 923.2132) -> (1823.1236, 669.2132)
  line L521 (1823.1236, 948.6132) -> (2077.1236, 948.6132)
  line L522 (2077.1236, 948.6132) -> (2077.1236, 1202.6132)
  line L523 (2077.1236, 1202.6132) -> (1823.1236, 1202.6132)
  line L524 (1823.1236, 1202.6132) -> (1823.1236, 948.6132)
  line L525 (1823.1236, 1228.0132) -> (2077.1236, 1228.0132)
  line L526 (2077.1236, 1228.0132) -> (2077.1236, 1482.0132)
  line L527 (2077.1236, 1482.0132) -> (1823.1236, 1482.0132)
  line L528 (1823.1236, 1482.0132) -> (1823.1236, 1228.0132)
  line L529 (1823.1236, 1507.4132) -> (2077.1236, 1507.4132)
  line L530 (2077.1236, 1507.4132) -> (2077.1236, 1761.4132)
  line L531 (2077.1236, 1761.4132) -> (1823.1236, 1761.4132)
  line L532 (1823.1236, 1761.4132) -> (1823.1236, 1507.4132)
  line L533 (1823.1236, 1786.8132) -> (2077.1236, 1786.8132)
  line L534 (2077.1236, 1786.8132) -> (2077.1236, 2040.8132)
  line L535 (2077.1236, 2040.8132) -> (1823.1236, 2040.8132)
  line L536 (1823.1236, 2040.8132) -> (1823.1236, 1786.8132)
  line L537 (1823.1236, 2066.2132) -> (2077.1236, 2066.2132)
  line L538 (2077.1236, 2066.2132) -> (2077.1236, 2320.2132)
  line L539 (2077.1236, 2320.2132) -> (1823.1236, 2320.2132)
  line L540 (1823.1236, 2320.2132) -> (1823.1236, 2066.2132)
  line L541 (1823.1236, 2345.6132) -> (2077.1236, 2345.6132)
  line L542 (2077.1236, 2345.6132) -> (2077.1236, 2599.6132)
  line L543 (2077.1236, 2599.6132) -> (1823.1236, 2599.6132)
  line L544 (1823.1236, 2599.6132) -> (1823.1236, 2345.6132)
  line L545 (1823.1236, 2625.0132) -> (2077.1236, 2625.0132)
  line L546 (2077.1236, 2625.0132) -> (2077.1236, 2879.0132)
  line L547 (2077.1236, 2879.0132) -> (1823.1236, 2879.0132)
  line L548 (1823.1236, 2879.0132) -> (1823.1236, 2625.0132)
  line L549 (1823.1236, 2904.4132) -> (2077.1236, 2904.4132)
  line L550 (2077.1236, 2904.4132) -> (2077.1236, 3158.4132)
  line L551 (2077.1236, 3158.4132) -> (1823.1236, 3158.4132)
  line L552 (1823.1236, 3158.4132) -> (1823.1236, 2904.4132)
  line L553 (1823.1236, 3183.8132) -> (2077.1236, 3183.8132)
  line L554 (2077.1236, 3183.8132) -> (2077.1236, 3437.8132)
  line L555 (2077.1236, 3437.8132) -> (1823.1236, 3437.8132)
  line L556 (1823.1236, 3437.8132) -> (1823.1236, 3183.8132)
  line L557 (1823.1236, 3463.2132) -> (2077.1236, 3463.2132)
  line L558 (2077.1236, 3463.2132) -> (2077.1236, 3717.2132)
  line L559 (2077.1236, 3717.2132) -> (1823.1236, 3717.2132)
  line L560 (1823.1236, 3717.2132) -> (1823.1236, 3463.2132)
  line L561 (1823.1236, 3742.6132) -> (2077.1236, 3742.6132)
  line L562 (2077.1236, 3742.6132) -> (2077.1236, 3996.6132)
  line L563 (2077.1236, 3996.6132) -> (1823.1236, 3996.6132)
  line L564 (1823.1236, 3996.6132) -> (1823.1236, 3742.6132)
  line L565 (1823.1236, 4022.0132) -> (2077.1236, 4022.0132)
  line L566 (2077.1236, 4022.0132) -> (2077.1236, 4276.0132)
  line L567 (2077.1236, 4276.0132) -> (1823.1236, 4276.0132)
  line L568 (1823.1236, 4276.0132) -> (1823.1236, 4022.0132)
  line L569 (1823.1236, 4301.4132) -> (2077.1236, 4301.4132)
  line L570 (2077.1236, 4301.4132) -> (2077.1236, 4555.4132)
  line L571 (2077.1236, 4555.4132) -> (1823.1236, 4555.4132)
  line L572 (1823.1236, 4555.4132) -> (1823.1236, 4301.4132)
  line L573 (1823.1236, 4580.8132) -> (2077.1236, 4580.8132)
  line L574 (2077.1236, 4580.8132) -> (2077.1236, 4834.8132)
  line L575 (2077.1236, 4834.8132) -> (1823.1236, 4834.8132)
  line L576 (1823.1236, 4834.8132) -> (1823.1236, 4580.8132)
  line L577 (1823.1236, 4860.2132) -> (2077.1236, 4860.2132)
  line L578 (2077.1236, 4860.2132) -> (2077.1236, 5114.2132)
  line L579 (2077.1236, 5114.2132) -> (1823.1236, 5114.2132)
  line L580 (1823.1236, 5114.2132) -> (1823.1236, 4860.2132)
  line L581 (1823.1236, 5139.6132) -> (2077.1236, 5139.6132)
  line L582 (2077.1236, 5139.6132) -> (2077.1236, 5393.6132)
  line L583 (2077.1236, 5393.6132) -> (1823.1236, 5393.6132)
  line L584 (1823.1236, 5393.6132) -> (1823.1236, 5139.6132)
  line L585 (1823.1236, 5419.0132) -> (2077.1236, 5419.0132)
  line L586 (2077.1236, 5419.0132) -> (2077.1236, 5673.0132)
  line L587 (2077.1236, 5673.0132) -> (1823.1236, 5673.0132)
  line L588 (1823.1236, 5673.0132) -> (1823.1236, 5419.0132)
  line L589 (1823.1236, 5698.4132) -> (2077.1236, 5698.4132)
  line L590 (2077.1236, 5698.4132) -> (2077.1236, 5952.4132)
  line L591 (2077.1236, 5952.4132) -> (1823.1236, 5952.4132)
  line L592 (1823.1236, 5952.4132) -> (1823.1236, 5698.4132)
  line L593 (2102.5236, 110.4132) -> (2356.5236, 110.4132)
  line L594 (2356.5236, 110.4132) -> (2356.5236, 364.4132)
  line L595 (2356.5236, 364.4132) -> (2102.5236, 364.4132)
  line L596 (2102.5236, 364.4132) -> (2102.5236, 110.4132)
  line L597 (2102.5236, 389.8132) -> (2356.5236, 389.8132)
  line L598 (2356.5236, 389.8132) -> (2356.5236, 643.8132)
  line L599 (2356.5236, 643.8132) -> (2102.5236, 643.8132)
  line L600 (2102.5236, 643.8132) -> (2102.5236, 389.8132)
  line L601 (2102.5236, 669.2132) -> (2356.5236, 669.2132)
  line L602 (2356.5236, 669.2132) -> (2356.5236, 923.2132)
  line L603 (2356.5236, 923.2132) -> (2102.5236, 923.2132)
  line L604 (2102.5236, 923.2132) -> (2102.5236, 669.2132)
  line L605 (2102.5236, 948.6132) -> (2356.5236, 948.6132)
  line L606 (2356.5236, 948.6132) -> (2356.5236, 1202.6132)
  line L607 (2356.5236, 1202.6132) -> (2102.5236, 1202.6132)
  line L608 (2102.5236, 1202.6132) -> (2102.5236, 948.6132)
  line L609 (2102.5236, 1228.0132) -> (2356.5236, 1228.0132)
  line L610 (2356.5236, 1228.0132) -> (2356.5236, 1482.0132)
  line L611 (2356.5236, 1482.0132) -> (2102.5236, 1482.0132)
  line L612 (2102.5236, 1482.0132) -> (2102.5236, 1228.0132)
  line L613 (2102.5236, 1507.4132) -> (2356.5236, 1507.4132)
  line L614 (2356.5236, 1507.4132) -> (2356.5236, 1761.4132)
  line L615 (2356.5236, 1761.4132) -> (2102.5236, 1761.4132)
  line L616 (2102.5236, 1761.4132) -> (2102.5236, 1507.4132)
  line L617 (2102.5236, 1786.8132) -> (2356.5236, 1786.8132)
  line L618 (2356.5236, 1786.8132) -> (2356.5236, 2040.8132)
  line L619 (2356.5236, 2040.8132) -> (2102.5236, 2040.8132)
  line L620 (2102.5236, 2040.8132) -> (2102.5236, 1786.8132)
  line L621 (2102.5236, 2066.2132) -> (2356.5236, 2066.2132)
  line L622 (2356.5236, 2066.2132) -> (2356.5236, 2320.2132)
  line L623 (2356.5236, 2320.2132) -> (2102.5236, 2320.2132)
  line L624 (2102.5236, 2320.2132) -> (2102.5236, 2066.2132)
  line L625 (2102.5236, 2345.6132) -> (2356.5236, 2345.6132)
  line L626 (2356.5236, 2345.6132) -> (2356.5236, 2599.6132)
  line L627 (2356.5236, 2599.6132) -> (2102.5236, 2599.6132)
  line L628 (2102.5236, 2599.6132) -> (2102.5236, 2345.6132)
  line L629 (2102.5236, 2625.0132) -> (2356.5236, 2625.0132)
  line L630 (2356.5236, 2625.0132) -> (2356.5236, 2879.0132)
  line L631 (2356.5236, 2879.0132) -> (2102.5236, 2879.0132)
  line L632 (2102.5236, 2879.0132) -> (2102.5236, 2625.0132)
  line L633 (2102.5236, 2904.4132) -> (2356.5236, 2904.4132)
  line L634 (2356.5236, 2904.4132) -> (2356.5236, 3158.4132)
  line L635 (2356.5236, 3158.4132) -> (2102.5236, 3158.4132)
  line L636 (2102.5236, 3158.4132) -> (2102.5236, 2904.4132)
  line L637 (2102.5236, 3183.8132) -> (2356.5236, 3183.8132)
  line L638 (2356.5236, 3183.8132) -> (2356.5236, 3437.8132)
  line L639 (2356.5236, 3437.8132) -> (2102.5236, 3437.8132)
  line L640 (2102.5236, 3437.8132) -> (2102.5236, 3183.8132)
  line L641 (2102.5236, 3463.2132) -> (2356.5236, 3463.2132)
  line L642 (2356.5236, 3463.2132) -> (2356.5236, 3717.2132)
  line L643 (2356.5236, 3717.2132) -> (2102.5236, 3717.2132)
  line L644 (2102.5236, 3717.2132) -> (2102.5236, 3463.2132)
  line L645 (2102.5236, 3742.6132) -> (2356.5236, 3742.6132)
  line L646 (2356.5236, 3742.6132) -> (2356.5236, 3996.6132)
  line L647 (2356.5236, 3996.6132) -> (2102.5236, 3996.6132)
  line L648 (2102.5236, 3996.6132) -> (2102.5236, 3742.6132)
  line L649 (2102.5236, 4022.0132) -> (2356.5236, 4022.0132)
  line L650 (2356.5236, 4022.0132) -> (2356.5236, 4276.0132)
  line L651 (2356.5236, 4276.0132) -> (2102.5236, 4276.0132)
  line L652 (2102.5236, 4276.0132) -> (2102.5236, 4022.0132)
  line L653 (2102.5236, 4301.4132) -> (2356.5236, 4301.4132)
  line L654 (2356.5236, 4301.4132) -> (2356.5236, 4555.4132)
  line L655 (2356.5236, 4555.4132) -> (2102.5236, 4555.4132)
  line L656 (2102.5236, 4555.4132) -> (2102.5236, 4301.4132)
  line L657 (2102.5236, 4580.8132) -> (2356.5236, 4580.8132)
  line L658 (2356.5236, 4580.8132) -> (2356.5236, 4834.8132)
  line L659 (2356.5236, 4834.8132) -> (2102.5236, 4834.8132)
  line L660 (2102.5236, 4834.8132) -> (2102.5236, 4580.8132)
  line L661 (2102.5236, 4860.2132) -> (2356.5236, 4860.2132)
  line L662 (2356.5236, 4860.2132) -> (2356.5236, 5114.2132)
  line L663 (2356.5236, 5114.2132) -> (2102.5236, 5114.2132)
  line L664 (2102.5236, 5114.2132) -> (2102.5236, 4860.2132)
  line L665 (2102.5236, 5139.6132) -> (2356.5236, 5139.6132)
  line L666 (2356.5236, 5139.6132) -> (2356.5236, 5393.6132)
  line L667 (2356.5236, 5393.6132) -> (2102.5236, 5393.6132)
  line L668 (2102.5236, 5393.6132) -> (2102.5236, 5139.6132)
  line L669 (2102.5236, 5419.0132) -> (2356.5236, 5419.0132)
  line L670 (2356.5236, 5419.0132) -> (2356.5236, 5673.0132)
  line L671 (2356.5236, 5673.0132) -> (2102.5236, 5673.0132)
  line L672 (2102.5236, 5673.0132) -> (2102.5236, 5419.0132)
  line L673 (2102.5236, 5698.4132) -> (2356.5236, 5698.4132)
  line L674 (2356.5236, 5698.4132) -> (2356.5236, 5952.4132)
  line L675 (2356.5236, 5952.4132) -> (2102.5236, 5952.4132)
  line L676 (2102.5236, 5952.4132) -> (2102.5236, 5698.4132)
  line L677 (2381.9236, 110.4132) -> (2635.9236, 110.4132)
  line L678 (2635.9236, 110.4132) -> (2635.9236, 364.4132)
  line L679 (2635.9236, 364.4132) -> (2381.9236, 364.4132)
  line L680 (2381.9236, 364.4132) -> (2381.9236, 110.4132)
  line L681 (2381.9236, 389.8132) -> (2635.9236, 389.8132)
  line L682 (2635.9236, 389.8132) -> (2635.9236, 643.8132)
  line L683 (2635.9236, 643.8132) -> (2381.9236, 643.8132)
  line L684 (2381.9236, 643.8132) -> (2381.9236, 389.8132)
  line L685 (2381.9236, 669.2132) -> (2635.9236, 669.2132)
  line L686 (2635.9236, 669.2132) -> (2635.9236, 923.2132)
  line L687 (2635.9236, 923.2132) -> (2381.9236, 923.2132)
  line L688 (2381.9236, 923.2132) -> (2381.9236, 669.2132)
  line L689 (2381.9236, 948.6132) -> (2635.9236, 948.6132)
  line L690 (2635.9236, 948.6132) -> (2635.9236, 1202.6132)
  line L691 (2635.9236, 1202.6132) -> (2381.9236, 1202.6132)
  line L692 (2381.9236, 1202.6132) -> (2381.9236, 948.6132)
  line L693 (2381.9236, 1228.0132) -> (2635.9236, 1228.0132)
  line L694 (2635.9236, 1228.0132) -> (2635.9236, 1482.0132)
  line L695 (2635.9236, 1482.0132) -> (2381.9236, 1482.0132)
  line L696 (2381.9236, 1482.0132) -> (2381.9236, 1228.0132)
  line L697 (2381.9236, 1507.4132) -> (2635.9236, 1507.4132)
  line L698 (2635.9236, 1507.4132) -> (2635.9236, 1761.4132)
  line L699 (2635.9236, 1761.4132) -> (2381.9236, 1761.4132)
  line L700 (2381.9236, 1761.4132) -> (2381.9236, 1507.4132)
  line L701 (2381.9236, 1786.8132) -> (2635.9236, 1786.8132)
  line L702 (2635.9236, 1786.8132) -> (2635.9236, 2040.8132)
  line L703 (2635.9236, 2040.8132) -> (2381.9236, 2040.8132)
  line L704 (2381.9236, 2040.8132) -> (2381.9236, 1786.8132)
  line L705 (2381.9236, 2066.2132) -> (2635.9236, 2066.2132)
  line L706 (2635.9236, 2066.2132) -> (2635.9236, 2320.2132)
  line L707 (2635.9236, 2320.2132) -> (2381.9236, 2320.2132)
  line L708 (2381.9236, 2320.2132) -> (2381.9236, 2066.2132)
  line L709 (2381.9236, 2345.6132) -> (2635.9236, 2345.6132)
  line L710 (2635.9236, 2345.6132) -> (2635.9236, 2599.6132)
  line L711 (2635.9236, 2599.6132) -> (2381.9236, 2599.6132)
  line L712 (2381.9236, 2599.6132) -> (2381.9236, 2345.6132)
  line L713 (2381.9236, 2625.0132) -> (2635.9236, 2625.0132)
  line L714 (2635.9236, 2625.0132) -> (2635.9236, 2879.0132)
  line L715 (2635.9236, 2879.0132) -> (2381.9236, 2879.0132)
  line L716 (2381.9236, 2879.0132) -> (2381.9236, 2625.0132)
  line L717 (2381.9236, 2904.4132) -> (2635.9236, 2904.4132)
  line L718 (2635.9236, 2904.4132) -> (2635.9236, 3158.4132)
  line L719 (2635.9236, 3158.4132) -> (2381.9236, 3158.4132)
  line L720 (2381.9236, 3158.4132) -> (2381.9236, 2904.4132)
  line L721 (2381.9236, 3183.8132) -> (2635.9236, 3183.8132)
  line L722 (2635.9236, 3183.8132) -> (2635.9236, 3437.8132)
  line L723 (2635.9236, 3437.8132) -> (2381.9236, 3437.8132)
  line L724 (2381.9236, 3437.8132) -> (2381.9236, 3183.8132)
  line L725 (2381.9236, 3463.2132) -> (2635.9236, 3463.2132)
  line L726 (2635.9236, 3463.2132) -> (2635.9236, 3717.2132)
  line L727 (2635.9236, 3717.2132) -> (2381.9236, 3717.2132)
  line L728 (2381.9236, 3717.2132) -> (2381.9236, 3463.2132)
  line L729 (2381.9236, 3742.6132) -> (2635.9236, 3742.6132)
  line L730 (2635.9236, 3742.6132) -> (2635.9236, 3996.6132)
  line L731 (2635.9236, 3996.6132) -> (2381.9236, 3996.6132)
  line L732 (2381.9236, 3996.6132) -> (2381.9236, 3742.6132)
  line L733 (2381.9236, 4022.0132) -> (2635.9236, 4022.0132)
  line L734 (2635.9236, 4022.0132) -> (2635.9236, 4276.0132)
  line L735 (2635.9236, 4276.0132) -> (2381.9236, 4276.0132)
  line L736 (2381.9236, 4276.0132) -> (2381.9236, 4022.0132)
  line L737 (2381.9236, 4301.4132) -> (2635.9236, 4301.4132)
  line L738 (2635.9236, 4301.4132) -> (2635.9236, 4555.4132)
  line L739 (2635.9236, 4555.4132) -> (2381.9236, 4555.4132)
  line L740 (2381.9236, 4555.4132) -> (2381.9236, 4301.4132)
  line L741 (2381.9236, 4580.8132) -> (2635.9236, 4580.8132)
  line L742 (2635.9236, 4580.8132) -> (2635.9236, 4834.8132)
  line L743 (2635.9236, 4834.8132) -> (2381.9236, 4834.8132)
  line L744 (2381.9236, 4834.8132) -> (2381.9236, 4580.8132)
  line L745 (2381.9236, 4860.2132) -> (2635.9236, 4860.2132)
  line L746 (2635.9236, 4860.2132) -> (2635.9236, 5114.2132)
  line L747 (2635.9236, 5114.2132) -> (2381.9236, 5114.2132)
  line L748 (2381.9236, 5114.2132) -> (2381.9236, 4860.2132)
  line L749 (2381.9236, 5139.6132) -> (2635.9236, 5139.6132)
  line L750 (2635.9236, 5139.6132) -> (2635.9236, 5393.6132)
  line L751 (2635.9236, 5393.6132) -> (2381.9236, 5393.6132)
  line L752 (2381.9236, 5393.6132) -> (2381.9236, 5139.6132)
  line L753 (2381.9236, 5419.0132) -> (2635.9236, 5419.0132)
  line L754 (2635.9236, 5419.0132) -> (2635.9236, 5673.0132)
  line L755 (2635.9236, 5673.0132) -> (2381.9236, 5673.0132)
  line L756 (2381.9236, 5673.0132) -> (2381.9236, 5419.0132)
  line L757 (2381.9236, 5698.4132) -> (2635.9236, 5698.4132)
  line L758 (2635.9236, 5698.4132) -> (2635.9236, 5952.4132)
  line L759 (2635.9236, 5952.4132) -> (2381.9236, 5952.4132)
  line L760 (2381.9236, 5952.4132) -> (2381.9236, 5698.4132)
  line L761 (2661.3236, 110.4132) -> (2915.3236, 110.4132)
  line L762 (2915.3236, 110.4132) -> (2915.3236, 364.4132)
  line L763 (2915.3236, 364.4132) -> (2661.3236, 364.4132)
  line L764 (2661.3236, 364.4132) -> (2661.3236, 110.4132)
  line L765 (2661.3236, 389.8132) -> (2915.3236, 389.8132)
  line L766 (2915.3236, 389.8132) -> (2915.3236, 643.8132)
  line L767 (2915.3236, 643.8132) -> (2661.3236, 643.8132)
  line L768 (2661.3236, 643.8132) -> (2661.3236, 389.8132)
  line L769 (2661.3236, 669.2132) -> (2915.3236, 669.2132)
  line L770 (2915.3236, 669.2132) -> (2915.3236, 923.2132)
  line L771 (2915.3236, 923.2132) -> (2661.3236, 923.2132)
  line L772 (2661.3236, 923.2132) -> (2661.3236, 669.2132)
  line L773 (2661.3236, 948.6132) -> (2915.3236, 948.6132)
  line L774 (2915.3236, 948.6132) -> (2915.3236, 1202.6132)
  line L775 (2915.3236, 1202.6132) -> (2661.3236, 1202.6132)
  line L776 (2661.3236, 1202.6132) -> (2661.3236, 948.6132)
  line L777 (2661.3236, 1228.0132) -> (2915.3236, 1228.0132)
  line L778 (2915.3236, 1228.0132) -> (2915.3236, 1482.0132)
  line L779 (2915.3236, 1482.0132) -> (2661.3236, 1482.0132)
  line L780 (2661.3236, 1482.0132) -> (2661.3236, 1228.0132)
  line L781 (2661.3236, 1507.4132) -> (2915.3236, 1507.4132)
  line L782 (2915.3236, 1507.4132) -> (2915.3236, 1761.4132)
  line L783 (2915.3236, 1761.4132) -> (2661.3236, 1761.4132)
  line L784 (2661.3236, 1761.4132) -> (2661.3236, 1507.4132)
  line L785 (2661.3236, 1786.8132) -> (2915.3236, 1786.8132)
  line L786 (2915.3236, 1786.8132) -> (2915.3236, 2040.8132)
  line L787 (2915.3236, 2040.8132) -> (2661.3236, 2040.8132)
  line L788 (2661.3236, 2040.8132) -> (2661.3236, 1786.8132)
  line L789 (2661.3236, 2066.2132) -> (2915.3236, 2066.2132)
  line L790 (2915.3236, 2066.2132) -> (2915.3236, 2320.2132)
  line L791 (2915.3236, 2320.2132) -> (2661.3236, 2320.2132)
  line L792 (2661.3236, 2320.2132) -> (2661.3236, 2066.2132)
  line L793 (2661.3236, 2345.6132) -> (2915.3236, 2345.6132)
  line L794 (2915.3236, 2345.6132) -> (2915.3236, 2599.6132)
  line L795 (2915.3236, 2599.6132) -> (2661.3236, 2599.6132)
  line L796 (2661.3236, 2599.6132) -> (2661.3236, 2345.6132)
  line L797 (2661.3236, 2625.0132) -> (2915.3236, 2625.0132)
  line L798 (2915.3236, 2625.0132) -> (2915.3236, 2879.0132)
  line L799 (2915.3236, 2879.0132) -> (2661.3236, 2879.0132)
  line L800 (2661.3236, 2879.0132) -> (2661.3236, 2625.0132)
  line L801 (2661.3236, 2904.4132) -> (2915.3236, 2904.4132)
  line L802 (2915.3236, 2904.4132) -> (2915.3236, 3158.4132)
  line L803 (2915.3236, 3158.4132) -> (2661.3236, 3158.4132)
  line L804 (2661.3236, 3158.4132) -> (2661.3236, 2904.4132)
  line L805 (2661.3236, 3183.8132) -> (2915.3236, 3183.8132)
  line L806 (2915.3236, 3183.8132) -> (2915.3236, 3437.8132)
  line L807 (2915.3236, 3437.8132) -> (2661.3236, 3437.8132)
  line L808 (2661.3236, 3437.8132) -> (2661.3236, 3183.8132)
  line L809 (2661.3236, 3463.2132) -> (2915.3236, 3463.2132)
  line L810 (2915.3236, 3463.2132) -> (2915.3236, 3717.2132)
  line L811 (2915.3236, 3717.2132) -> (2661.3236, 3717.2132)
  line L812 (2661.3236, 3717.2132) -> (2661.3236, 3463.2132)
  line L813 (2661.3236, 3742.6132) -> (2915.3236, 3742.6132)
  line L814 (2915.3236, 3742.6132) -> (2915.3236, 3996.6132)
  line L815 (2915.3236, 3996.6132) -> (2661.3236, 3996.6132)